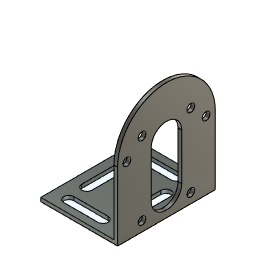
Motor mounting v2 (Autodesk Fusion 360 design; units mm, degrees)
Autodesk Fusion 360 part; units mm, degrees
sketch "Sketch1" plane through (0, 0, 0) normal (1, 0, 0) x (0, 1, 0)
  line L0 (20, -24) -> (-20, -24)
  line L1 (-20, -24) -> (-20, 4)
  line L2 (20, 4) -> (20, -24)
  arc A0 (20, 4) -> (-20, 4) centre (0, 4) ccw
  line L3 (-6.25, 4) -> (-6.25, -15)
  arc A1 (-6.25, -15) -> (6.25, -15) centre (0, -15) ccw
  line L4 (6.25, -15) -> (6.25, 4)
  arc A2 (6.25, 4) -> (-6.25, 4) centre (0, 4) ccw
  line L5 (0, 4) -> (0, -15) construction
  circle A3 centre (-16.237, 4) radius 1.6
  circle A4 centre (-10, -20) radius 1.6
  circle A5 centre (10, -20) radius 1.6
  circle A6 centre (-10, 10) radius 1.6
  circle A7 centre (10, 10) radius 1.6
  circle A8 centre (16.237, 4) radius 1.6
  dimension "d4" = 12.5
  dimension "d5" = 3.2
  dimension "d6" = 3.2
  dimension "d9" = 20
  dimension "d10" = 30
  constraint horizontal L0
  constraint perpendicular L0 L1
  constraint parallel L1 L2
  constraint tangent L2 A0
  constraint tangent L3 A1
  constraint tangent A1 L4
  constraint parallel L3 L4
  constraint tangent L4 A2
  constraint tangent L3 A2
  constraint parallel L1 L5
  constraint coincident A0.centre A2.centre
  constraint symmetric L5 A3 A8
  measures "d4" diameter of A1
  measures "d5" diameter of A3
  measures "d6" diameter of A4
extrude "Extrude1" add sketch "Sketch1" along normal blind 1.5
sketch "Sketch2" plane through (0, 0, 0) normal (-1, 0, 0) x (0, -1, 0)
  circle A0 centre (10, 10) radius 1.6
  circle A1 centre (-10, 10) radius 1.6
  circle A2 centre (-16.237, 4) radius 1.6
  circle A3 centre (10, -20) radius 1.6
  circle A4 centre (-10, -20) radius 1.6
  circle A5 centre (16.237, 4) radius 1.6
  arc A6 (6.25, 4) -> (-6.25, 4) centre (0, 4) ccw
  line L0 (6.25, 4) -> (6.25, -15)
  arc A7 (-6.25, -15) -> (6.25, -15) centre (0, -15) ccw
  line L1 (-6.25, -15) -> (-6.25, 4)
  line L2 (-20, 4) -> (-20, -24)
  line L3 (-20, -24) -> (20, -24)
  line L4 (20, -24) -> (20, 4)
  arc A8 (20, 4) -> (-20, 4) centre (0, 4) ccw
  line L5 (-20, -24) -> (20, -24)
  line L6 (20, -24) -> (20, -22.5)
  line L7 (20, -22.5) -> (-20, -22.5)
  line L8 (-20, -22.5) -> (-20, -24)
  dimension "d13" = 1.5
  constraint horizontal L5
  constraint vertical L6
  constraint horizontal L7
  constraint vertical L8
  constraint coincident L2.end L3.start
  measures "d13" distance of L2.end L7.end
extrude "Extrude2" add sketch "Sketch2" along normal blind 30 contours L2 L3 L4 L5 L6 L7 L8
sketch "Sketch3" plane through (0, 0, -22.5) normal (0, 0, 1) x (-1, 0, 0)
  line L0 (0, 20) -> (0, -20)
  line L1 (0, -20) -> (30, -20)
  line L2 (30, -20) -> (30, 20)
  line L3 (30, 20) -> (0, 20)
sketch "Sketch4" plane through (0, 0, -22.5) normal (0, 0, 1) x (1, 0, 0)
  line L0 (-23.5, 12.9) -> (-9.5, 12.9)
  arc A0 (-9.5, 12.9) -> (-9.5, 17.1) centre (-9.5, 15) ccw
  line L1 (-9.5, 17.1) -> (-23.5, 17.1)
  arc A1 (-23.5, 17.1) -> (-23.5, 12.9) centre (-23.5, 15) ccw
  line L2 (-23.5, 15) -> (-9.5, 15) construction
  line L3 (-23.5, -12.9) -> (-9.5, -12.9)
  arc A2 (-23.5, -12.9) -> (-23.5, -17.1) centre (-23.5, -15) ccw
  line L4 (-9.5, -17.1) -> (-23.5, -17.1)
  arc A3 (-9.5, -17.1) -> (-9.5, -12.9) centre (-9.5, -15) ccw
  line L5 (-26.2852, 7.0901) -> (-26.2852, -6.9099)
  arc A4 (-26.2852, -6.9099) -> (-22.0852, -6.9099) centre (-24.1852, -6.9099) ccw
  line L6 (-22.0852, -6.9099) -> (-22.0852, 7.0901)
  arc A5 (-22.0852, 7.0901) -> (-26.2852, 7.0901) centre (-24.1852, 7.0901) ccw
  line L7 (-24.1852, 7.0901) -> (-24.1852, -6.9099) construction
  line L8 (-7.9148, -6.9099) -> (-7.9148, 7.0901)
  arc A6 (-3.7148, 7.0901) -> (-7.9148, 7.0901) centre (-5.8148, 7.0901) ccw
  line L9 (-3.7148, 7.0901) -> (-3.7148, -6.9099)
  arc A7 (-7.9148, -6.9099) -> (-3.7148, -6.9099) centre (-5.8148, -6.9099) ccw
  dimension "d17" = 14
  dimension "d18" = 4.2
  dimension "d19" = 4.2
  constraint tangent L0 A0
  constraint tangent A0 L1
  constraint parallel L0 L1
  constraint tangent L1 A1
  constraint tangent L0 A1
  constraint tangent L5 A4
  constraint tangent A4 L6
  constraint parallel L5 L6
  constraint tangent L6 A5
  constraint tangent L5 A5
  constraint vertical L7
  measures "d17" distance of A1.centre A0.centre
  measures "d18" diameter of A0
  measures "d19" diameter of A4
extrude "Extrude3" cut sketch "Sketch4" against normal blind 1.5
